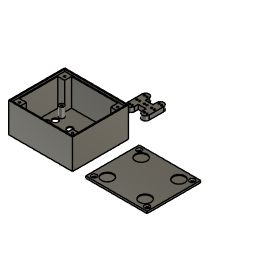
dice (Autodesk Fusion 360 design; units mm, degrees)
Autodesk Fusion 360 part; units mm, degrees
note: some values were not read from the file. Set by a fixed rule: which face or edge a step refers to.
sketch "Sketch1" plane through (0, 0, 0) normal (0, 0, 1) x (1, 0, 0)
  line L0 (0, 0) -> (61, 0)
  line L1 (61, 0) -> (61, -53)
  line L2 (61, -53) -> (0, -53)
  line L3 (0, -53) -> (0, 0)
  line L4 (-1, 1) -> (62, 1)
  line L5 (62, 1) -> (62, -54)
  line L6 (62, -54) -> (-1, -54)
  line L7 (-1, -54) -> (-1, 1)
  line L8 (-2, 2) -> (63, 2)
  line L9 (63, 2) -> (63, -55)
  line L10 (63, -55) -> (-2, -55)
  line L11 (-2, -55) -> (-2, 2)
  line L12 (0, -53) -> (7, -53)
  line L13 (7, -53) -> (7, -46)
  line L14 (7, -46) -> (0, -46)
  line L15 (0, -46) -> (0, -53)
  line L16 (61, -53) -> (54, -53)
  line L17 (54, -53) -> (54, -46)
  line L18 (54, -46) -> (61, -46)
  line L19 (61, -46) -> (61, -53)
  line L20 (61, 0) -> (54, 0)
  line L21 (54, 0) -> (54, -7)
  line L22 (54, -7) -> (61, -7)
  line L23 (61, -7) -> (61, 0)
  line L24 (0, 0) -> (7, 0)
  line L25 (7, 0) -> (7, -7)
  line L26 (7, -7) -> (0, -7)
  line L27 (0, -7) -> (0, 0)
  line L28 (61, 0) -> (53.5, 0)
  line L29 (61, -26.5) -> (61, 0)
  line L30 (61, 0) -> (43.5, 0)
  line L31 (61, -26.5) -> (61, 0)
  circle A0 centre (43.5, -26.5) radius 4
  circle A1 centre (53.5, -26.5) radius 3.5
  line L32 (61, -53) -> (42.5, -53)
  line L33 (61, -34.5) -> (61, -53)
  circle A2 centre (42.5, -34.5) radius 2.5
  line L34 (0, -53) -> (16.5, -53)
  line L35 (0, -34.5) -> (0, -53)
  circle A3 centre (16.5, -34.5) radius 2.5
  line L36 (0, 0) -> (9.5, 0)
  line L37 (0, -12.5) -> (0, 0)
  circle A4 centre (9.5, -12.5) radius 2.5
  line L38 (61, 0) -> (55.5, 0)
  line L39 (61, -19.5) -> (61, 0)
  circle A5 centre (55.5, -19.5) radius 2.5
  line L40 (0, 0) -> (9.5, 0)
  line L41 (0, -26.5) -> (0, 0)
  circle A6 centre (9.5, -19) radius 3
  circle A7 centre (9.5, -26.5) radius 3
  circle A8 centre (9.5, -34) radius 3
  circle A9 centre (17, -26.5) radius 3
  circle A10 centre (24.5, -19) radius 3
  circle A11 centre (24.5, -26.5) radius 3
  circle A12 centre (24.5, -34) radius 3
  dimension "d1" = 61
  dimension "d2" = 53
  dimension "d3" = 63
  dimension "d4" = 55
  dimension "d5" = 65
  dimension "d6" = 57
  dimension "d7" = 7
  dimension "d8" = 7
  dimension "d9" = 7
  dimension "d10" = 7
  dimension "d11" = 7
  dimension "d12" = 7
  dimension "d13" = 7
  dimension "d14" = 7
  dimension "d15" = 7.5
  dimension "d16" = 26.5
  dimension "d17" = 17.5
  dimension "d18" = 8
  dimension "d19" = 7
  dimension "d20" = 18.5
  dimension "d21" = 18.5
  dimension "d22" = 5
  dimension "d23" = 16.5
  dimension "d24" = 18.5
  dimension "d25" = 5
  dimension "d26" = 9.5
  dimension "d27" = 12.5
  dimension "d28" = 5
  dimension "d29" = 5.5
  dimension "d30" = 19.5
  dimension "d31" = 5
  dimension "d32" = 9.5
  dimension "d33" = 26.5
  dimension "d34" = 7.5
  dimension "d35" = 7.5
  dimension "d39" = 7.5
  dimension "d42" = 6
  dimension "d43" = 6
  dimension "d44" = 6
  dimension "d45" = 6
  dimension "d46" = 6
  dimension "d47" = 6
  dimension "d48" = 6
  constraint horizontal L0
  constraint vertical L1
  constraint horizontal L2
  constraint vertical L3
  constraint coincident L0.start L3.end
  constraint horizontal L4
  constraint vertical L5
  constraint horizontal L6
  constraint vertical L7
  constraint horizontal L8
  constraint vertical L9
  constraint horizontal L10
  constraint vertical L11
  constraint horizontal L12
  constraint vertical L13
  constraint horizontal L14
  constraint vertical L15
  constraint horizontal L16
  constraint vertical L17
  constraint horizontal L18
  constraint vertical L19
  constraint horizontal L20
  constraint vertical L21
  constraint horizontal L22
  constraint vertical L23
  constraint horizontal L24
  constraint vertical L25
  constraint horizontal L26
  constraint vertical L27
  constraint horizontal L28
  constraint vertical L29
  constraint horizontal L30
  constraint vertical L31
  constraint horizontal L32
  constraint vertical L33
  constraint horizontal L34
  constraint vertical L35
  constraint horizontal L36
  constraint vertical L37
  constraint horizontal L38
  constraint vertical L39
  constraint horizontal L40
  constraint vertical L41
  measures "d1" distance of L0.start L0.end
  measures "d2" distance of L0.start L2.end
  measures "d3" distance of L4.start L4.end
  measures "d4" distance of L4.start L6.end
  measures "d5" distance of L8.start L8.end
  measures "d6" distance of L8.start L10.end
  measures "d7" distance of L2.end L12.end
  measures "d8" distance of L2.end L14.end
  measures "d9" distance of L1.end L16.end
  measures "d10" distance of L1.end L18.end
  measures "d11" distance of L0.end L20.end
  measures "d12" distance of L0.end L22.end
  measures "d13" distance of L0.start L24.end
  measures "d14" distance of L0.start L26.end
  measures "d15" distance of L0.end L28.end
  measures "d16" distance of L0.end L29.start
  measures "d17" distance of L0.end L30.end
  measures "d18" diameter of A0
  measures "d19" diameter of A1
  measures "d20" distance of L1.end L32.end
  measures "d21" distance of L1.end L33.start
  measures "d22" diameter of A2
  measures "d23" distance of L2.end L34.end
  measures "d24" distance of L2.end L35.start
  measures "d25" diameter of A3
  measures "d26" distance of L0.start L36.end
  measures "d27" distance of L0.start L37.start
  measures "d28" diameter of A4
  measures "d29" distance of L0.end L38.end
  measures "d30" distance of L0.end L39.start
  measures "d31" diameter of A5
  measures "d32" distance of L0.start L36.end
  measures "d33" distance of L0.start L41.start
  measures "d34" distance of A7.centre A9.centre
  measures "d35" distance of A6.centre A7.centre
  measures "d39" distance of A7.centre A8.centre
  measures "d42" diameter of A6
  measures "d43" diameter of A7
  measures "d44" diameter of A8
  measures "d45" diameter of A9
  measures "d46" diameter of A10
  measures "d47" diameter of A11
  measures "d48" diameter of A12
extrude "Extrude1" add sketch "Sketch1" along normal blind 1 contours L0 L1 L2 L3 L13 L14 L17 L18 L21 L22 L25 L26 L28 L29 L30 L31 L32 L33 L34 L35 L36 L37 L39 L40 L41 makes body 1
extrude "Extrude2" add sketch "Sketch1" along normal blind 11 contours A2 | A3 | A4 | A5 bodies 1
extrude "Extrude3" add sketch "Sketch1" along normal blind 30 contours L0 L3 L24 L25 L26 L27 L36 L37 L40 L41 | L0 L1 L20 L21 L22 L23 L28 L29 L30 L31 L38 L39 | L2 L3 L12 L13 L14 L15 L34 L35 | L1 L2 L16 L17 L18 L19 L32 L33 | L4 L5 L6 L7 bodies 1
extrude "Extrude4" add sketch "Sketch1" along normal blind 31 contours L8 L9 L10 L11 bodies 1
sketch "Sketch2" plane through (0, 0, 11) normal (0, 0, 1) x (-1, 0, 0)
  circle A0 centre (-9.5, 12.5) radius 2.5
  circle A1 centre (-9.5, 12.5) radius 0.9
  circle A2 centre (-16.5, 34.5) radius 0.9
  circle A3 centre (-42.5, 34.5) radius 0.9
  circle A4 centre (-55.5, 19.5) radius 0.9
  dimension "d57" = 1.8
  dimension "d58" = 1.8
  dimension "d59" = 1.8
  dimension "d60" = 1.8
  constraint concentric A0 A1
  measures "d57" diameter of A1
  measures "d58" diameter of A2
  measures "d59" diameter of A3
  measures "d60" diameter of A4
extrude "Extrude5" cut sketch "Sketch2" against normal blind 7 contours A1 | A2 | A3 | A4 bodies 1
sketch "Sketch3" plane through (0, 0, 30) normal (0, 0, 1) x (-1, 0, 0)
  line L0 (0, 46) -> (0, 7)
  line L1 (0, 7) -> (-7, 7)
  line L2 (-7, 7) -> (-7, 0)
  line L3 (-7, 0) -> (-54, 0)
  line L4 (-54, 0) -> (-54, 7)
  line L5 (-54, 7) -> (-61, 7)
  line L6 (-61, 7) -> (-61, 46)
  line L7 (-61, 46) -> (-54, 46)
  line L8 (-54, 46) -> (-54, 53)
  line L9 (-54, 53) -> (-7, 53)
  line L10 (-7, 53) -> (-7, 46)
  line L11 (-7, 46) -> (0, 46)
  line L12 (1, 54) -> (-62, 54)
  line L13 (-62, 54) -> (-62, -1)
  line L14 (-62, -1) -> (1, -1)
  line L15 (1, -1) -> (1, 54)
  line L16 (1, -1) -> (-3.5, -1)
  line L17 (1, 3.5) -> (1, -1)
  circle A0 centre (-3.5, 3.5) radius 1
  line L18 (1, 54) -> (-3.5, 54)
  line L19 (1, 49.5) -> (1, 54)
  circle A1 centre (-3.5, 49.5) radius 1
  line L20 (-62, 54) -> (-57.5, 54)
  line L21 (-62, 49.5) -> (-62, 54)
  circle A2 centre (-57.5, 49.5) radius 1
  line L22 (-62, -1) -> (-57.5, -1)
  line L23 (-62, 3.5) -> (-62, -1)
  circle A3 centre (-57.5, 3.5) radius 1
  dimension "d63" = 2
  dimension "d64" = 4.5
  dimension "d65" = 4.5
  dimension "d66" = 2
  dimension "d67" = 4.5
  dimension "d68" = 4.5
  dimension "d69" = 2
  dimension "d70" = 4.5
  dimension "d71" = 4.5
  dimension "d72" = 2
  constraint horizontal L16
  constraint vertical L17
  constraint coincident L14.end L15.start
  constraint horizontal L18
  constraint vertical L19
  constraint coincident L12.start L15.end
  constraint horizontal L20
  constraint vertical L21
  constraint coincident L12.end L13.start
  constraint horizontal L22
  constraint vertical L23
  constraint coincident L13.end L14.start
  measures "d63" diameter of A0
  measures "d64" distance of L12.start L18.end
  measures "d65" distance of L12.start L19.start
  measures "d66" diameter of A1
  measures "d67" distance of L12.end L20.end
  measures "d68" distance of L12.end L21.start
  measures "d69" diameter of A2
  measures "d70" distance of L13.end L22.end
  measures "d71" distance of L13.end L23.start
  measures "d72" diameter of A3
extrude "Extrude6" cut sketch "Sketch3" against normal blind 12 contours A0 | A1 | A2 | A3 bodies 1
sketch "Sketch4" plane through (0, 0, 0) normal (0, 0, 1) x (1, 0, 0)
  line L0 (75, 1) -> (137.5, 1)
  line L1 (137.5, 1) -> (137.5, -53.5)
  line L2 (137.5, -53.5) -> (75, -53.5)
  line L3 (75, -53.5) -> (75, 1)
  line L4 (75, 1) -> (79.25, 1)
  line L5 (75, -3.25) -> (75, 1)
  circle A0 centre (79.25, -3.25) radius 1.4
  line L6 (75, -53.5) -> (79.25, -53.5)
  line L7 (75, -49.25) -> (75, -53.5)
  circle A1 centre (79.25, -49.25) radius 1.4
  line L8 (137.5, -53.5) -> (133.25, -53.5)
  line L9 (137.5, -49.25) -> (137.5, -53.5)
  circle A2 centre (133.25, -49.25) radius 1.4
  line L10 (137.5, 1) -> (133.25, 1)
  line L11 (137.5, -3.25) -> (137.5, 1)
  circle A3 centre (133.25, -3.25) radius 1.4
  line L12 (75, 1) -> (87, 1)
  line L13 (75, -9) -> (75, 1)
  line L14 (137.5, 1) -> (125.5, 1)
  line L15 (137.5, -9) -> (137.5, 1)
  line L16 (137.5, -53.5) -> (125.5, -53.5)
  line L17 (137.5, -43.5) -> (137.5, -53.5)
  line L18 (75, -53.5) -> (87, -53.5)
  line L19 (75, -43.5) -> (75, -53.5)
  dimension "d75" = 62.5
  dimension "d76" = 54.5
  dimension "d83" = 4.25
  dimension "d84" = 4.25
  dimension "d85" = 2.8
  dimension "d86" = 4.25
  dimension "d87" = 4.25
  dimension "d88" = 2.8
  dimension "d89" = 4.25
  dimension "d90" = 4.25
  dimension "d91" = 2.8
  dimension "d92" = 4.25
  dimension "d93" = 4.25
  dimension "d94" = 2.8
  constraint horizontal L0
  constraint vertical L1
  constraint horizontal L2
  constraint vertical L3
  constraint horizontal L4
  constraint vertical L5
  constraint horizontal L6
  constraint vertical L7
  constraint horizontal L8
  constraint vertical L9
  constraint horizontal L10
  constraint vertical L11
  constraint horizontal L12
  constraint vertical L13
  constraint horizontal L14
  constraint vertical L15
  constraint horizontal L16
  constraint vertical L17
  constraint horizontal L18
  constraint vertical L19
  measures "d75" distance of L0.start L0.end
  measures "d76" distance of L0.start L2.end
  measures "d83" distance of L0.start L4.end
  measures "d84" distance of L0.start L5.start
  measures "d85" diameter of A0
  measures "d86" distance of L2.end L6.end
  measures "d87" distance of L2.end L7.start
  measures "d88" diameter of A1
  measures "d89" distance of L1.end L8.end
  measures "d90" distance of L1.end L9.start
  measures "d91" diameter of A2
  measures "d92" distance of L0.end L10.end
  measures "d93" distance of L0.end L11.start
  measures "d94" diameter of A3
extrude "Extrude7" cut 1 faces at (3.1391, -0.5011, 30) along direction (0, 0, -1) blind 1 on bodies 1 bodies 1
extrude "Extrude8" add sketch "Sketch1" along normal blind 30 contours L4 L5 L6 L7 bodies 1
extrude "Extrude9" add 4 faces at (3.4751, -0.8343, 29) (57.5249, -6.1657, 29) (57.5249, -52.1657, 29) (3.5249, -52.1657, 29) along direction (0, 0, 1) blind 1 on bodies 1 bodies 1
extrude "Extrude10" cut 1 faces at (3.1391, -0.5011, 30) along direction (0, 0, -1) blind 1 on bodies 1 bodies 1
extrude "Extrude11" add sketch "Sketch4" along normal blind 2 separate body makes body 2
chamfer "Chamfer1" distance 1.2 angle 45 4 edges at (77.9447, -2.7437, 2) (77.9447, -48.7437, 2) (131.9447, -48.7437, 2) (131.9447, -2.7437, 2) on bodies 2
sketch "Sketch5" plane through (0, 0, 2) normal (0, 0, 1) x (-1, 0, 0)
  circle A0 centre (-133.25, 49.25) radius 2.6
  circle A1 centre (-79.25, 3.25) radius 2.6
  line L0 (-75, -1) -> (-75, 53.5)
  line L1 (-75, 53.5) -> (-137.5, 53.5)
  line L2 (-137.5, 53.5) -> (-137.5, -1)
  line L3 (-137.5, -1) -> (-75, -1)
  circle A2 centre (-79.25, 49.25) radius 2.6
  circle A3 centre (-133.25, 3.25) radius 2.6
  line L4 (-75, -1) -> (-87, -1)
  line L5 (-75, 9) -> (-75, -1)
  circle A4 centre (-87, 9) radius 6
  line L6 (-137.5, -1) -> (-125.5, -1)
  line L7 (-137.5, 9) -> (-137.5, -1)
  circle A5 centre (-125.5, 9) radius 6
  line L8 (-137.5, 53.5) -> (-125.5, 53.5)
  line L9 (-137.5, 43.5) -> (-137.5, 53.5)
  circle A6 centre (-125.5, 43.5) radius 6
  line L10 (-75, 53.5) -> (-87, 53.5)
  line L11 (-75, 43.5) -> (-75, 53.5)
  circle A7 centre (-87, 43.5) radius 6
  dimension "d114" = 12
  dimension "d115" = 10
  dimension "d116" = 12
  dimension "d117" = 12
  dimension "d118" = 10
  dimension "d119" = 12
  dimension "d120" = 12
  dimension "d121" = 10
  dimension "d122" = 12
  dimension "d123" = 12
  dimension "d124" = 10
  dimension "d125" = 12
  constraint horizontal L4
  constraint vertical L5
  constraint coincident L0.start L3.end
  constraint horizontal L6
  constraint vertical L7
  constraint coincident L2.end L3.start
  constraint horizontal L8
  constraint vertical L9
  constraint coincident L1.end L2.start
  constraint horizontal L10
  constraint vertical L11
  constraint coincident L0.end L1.start
  measures "d114" distance of L0.start L4.end
  measures "d115" distance of L0.start L5.start
  measures "d116" diameter of A4
  measures "d117" distance of L2.end L6.end
  measures "d118" distance of L2.end L7.start
  measures "d119" diameter of A5
  measures "d120" distance of L1.end L8.end
  measures "d121" distance of L1.end L9.start
  measures "d122" diameter of A6
  measures "d123" distance of L0.end L10.end
  measures "d124" distance of L0.end L11.start
  measures "d125" diameter of A7
extrude "Extrude12" cut sketch "Sketch5" against normal blind 0.8 contours A4 | A5 | A6 | A7 bodies 2
sketch "Sketch6" plane through (0, 0, 0) normal (0, 0, 1) x (1, 0, 0)
  circle A0 centre (5, 10) radius 3.5
  circle A1 centre (15, 10) radius 3
  dimension "d128" = 7
  dimension "d135" = 6
  measures "d128" diameter of A0
  measures "d135" diameter of A1
extrude "Extrude13" add sketch "Sketch6" along normal blind 8 separate body contours A0 makes body 3
sketch "Sketch7" plane through (0, 0, 8) normal (0, 0, 1) x (-1, 0, 0)
  circle A0 centre (-5, -10) radius 3.5
  circle A1 centre (-5, -10) radius 1.75
  dimension "d131" = 3.5
  constraint concentric A0 A1
  measures "d131" diameter of A1
extrude "Extrude15" add sketch "Sketch6" along normal blind 3.5 separate body contours A1 makes body 4
chamfer "Chamfer3" distance 0.6 angle 45 1 edges at (12.203, 8.9152, 0) on bodies 4
chamfer "Chamfer4" distance 0.6 angle 45 1 edges at (1.7369, 8.7343, 0) on bodies 3
sketch "Sketch8" plane through (0, 0, 3.5) normal (0, 0, 1) x (-1, 0, 0)
  circle A0 centre (-15, -10) radius 3
  line L0 (-13.3, -11.2) -> (-16.7, -11.2)
  line L1 (-16.7, -11.2) -> (-16.7, -8.8)
  line L2 (-16.7, -8.8) -> (-13.3, -8.8)
  line L3 (-13.3, -8.8) -> (-13.3, -11.2)
  dimension "d140" = 3.4
  dimension "d141" = 2.4
  constraint horizontal L0
  constraint vertical L1
  constraint horizontal L2
  constraint vertical L3
  measures "d140" distance of L0.start L0.end
  measures "d141" distance of L0.start L2.end
extrude "Extrude16" cut sketch "Sketch8" against normal blind 2.5 contours L0 L1 L2 L3 bodies 4
extrude "Extrude17" cut sketch "Sketch7" against normal blind 3.5 contours A1 bodies 3
chamfer "Chamfer5" distance 0.6 angle 45 4 edges at (30.5, 2, 0) (-2, -26.5, 0) (30.5, -55, 0) (63, -26.5, 0) on bodies 1
sketch "Sketch9" plane through (0, 0, 0) normal (0, 0, 1) x (1, 0, 0)
  circle A0 centre (37.5129, 45) radius 3
  circle A1 centre (37.5129, 37.5) radius 3
  circle A2 centre (37.5129, 30) radius 3
  circle A3 centre (45.0129, 37.5) radius 3
  circle A4 centre (52.5129, 37.5) radius 3
  circle A5 centre (52.5, 45) radius 3
  circle A6 centre (52.5, 30) radius 3
  circle A7 centre (37.5129, 45) radius 3.6
  circle A8 centre (37.5129, 37.5) radius 3.6
  circle A9 centre (37.5129, 30) radius 3.6
  circle A10 centre (45.0129, 37.5) radius 3.6
  circle A11 centre (52.5, 45) radius 3.6
  circle A12 centre (52.5129, 37.5) radius 3.6
  circle A13 centre (52.5, 30) radius 3.6
  line L0 (33.9129, 44.9997) -> (33.9129, 30)
  line L1 (48.9, 30.0018) -> (48.9, 33.9)
  line L2 (48.9, 33.9) -> (41.1129, 33.9)
  line L3 (41.1129, 33.9) -> (41.1129, 30.0018)
  line L4 (48.9, 45.0043) -> (48.9, 41.1)
  line L5 (48.9, 41.1) -> (41.1129, 41.1)
  line L6 (41.1129, 41.1) -> (41.1129, 45.0043)
  line L7 (56.1, 45) -> (56.1, 30)
  circle A14 centre (38.8, 45) radius 0.9
  circle A15 centre (36.2, 45) radius 0.9
  circle A16 centre (38.8, 37.5) radius 0.9
  circle A17 centre (36.2, 37.5) radius 0.9
  circle A18 centre (38.8, 30) radius 0.9
  circle A19 centre (36.2, 30) radius 0.9
  circle A20 centre (46.3, 37.5) radius 0.9
  circle A21 centre (43.7, 37.5) radius 0.9
  circle A22 centre (53.8, 45) radius 0.9
  circle A23 centre (51.2, 45) radius 0.9
  circle A24 centre (53.8, 37.5) radius 0.9
  circle A25 centre (51.2, 37.5) radius 0.9
  circle A26 centre (53.8, 30) radius 0.9
  circle A27 centre (51.2, 30) radius 0.9
  line L8 (34.6629, 49.5) -> (34.6629, 25)
  line L9 (42.1629, 42) -> (42.1629, 33)
  line L10 (49.65, 50) -> (49.65, 25)
  dimension "d147" = 6
  dimension "d148" = 6
  dimension "d149" = 7.5
  dimension "d150" = 6
  dimension "d151" = 7.5
  dimension "d152" = 6
  dimension "d153" = 7.5
  dimension "d154" = 7.5
  dimension "d155" = 6
  dimension "d156" = 7.5
  dimension "d157" = 7.5
  dimension "d158" = 6
  dimension "d159" = 6
  dimension "d160" = 7.2
  dimension "d161" = 7.2
  dimension "d162" = 7.2
  dimension "d163" = 7.2
  dimension "d164" = 7.2
  dimension "d165" = 7.2
  dimension "d166" = 7.2
  dimension "d167" = 1.8
  dimension "d168" = 1.8
  dimension "d169" = 2.6
  dimension "d170" = 1.8
  dimension "d171" = 1.8
  dimension "d172" = 1.8
  dimension "d173" = 1.8
  dimension "d174" = 1.8
  dimension "d175" = 1.8
  dimension "d176" = 1.8
  dimension "d177" = 1.8
  dimension "d178" = 1.8
  dimension "d179" = 1.8
  dimension "d180" = 1.8
  dimension "d181" = 1.8
  dimension "d182" = 2.85
  dimension "d183" = 2.85
  dimension "d184" = 14.9871
  dimension "d185" = 2.85
  constraint concentric A0 A7
  constraint concentric A1 A8
  constraint concentric A2 A9
  constraint concentric A3 A10
  constraint concentric A5 A11
  constraint concentric A4 A12
  constraint concentric A6 A13
  constraint coincident A7 L0.start
  constraint coincident A9 L0.end
  constraint tangent A9 L0
  constraint vertical L1
  constraint horizontal L2
  constraint vertical L3
  constraint coincident A9 L3.end
  constraint vertical L4
  constraint horizontal L5
  constraint vertical L6
  constraint coincident A7 L6.end
  constraint coincident A11 L7.start
  constraint coincident A13 L7.end
  constraint tangent A13 L7
  constraint parallel L0 L8
  constraint perpendicular L5 L9
  constraint vertical L10
  measures "d147" diameter of A0
  measures "d148" diameter of A1
  measures "d149" distance of A0.centre A1.centre
  measures "d150" diameter of A2
  measures "d151" distance of A1.centre A2.centre
  measures "d152" diameter of A3
  measures "d153" horizontal distance of A1.centre A3.centre
  measures "d154" vertical distance of A0.centre A3.centre
  measures "d155" diameter of A4
  measures "d156" horizontal distance of A3.centre A4.centre
  measures "d157" vertical distance of A0.centre A4.centre
  measures "d158" diameter of A5
  measures "d159" diameter of A6
  measures "d160" diameter of A7
  measures "d161" diameter of A8
  measures "d162" diameter of A9
  measures "d163" diameter of A10
  measures "d164" diameter of A11
  measures "d165" diameter of A12
  measures "d166" diameter of A13
  measures "d167" diameter of A14
  measures "d168" diameter of A15
  measures "d169" distance of A14.centre A15.centre
  measures "d170" diameter of A16
  measures "d171" diameter of A17
  measures "d172" diameter of A18
  measures "d173" diameter of A19
  measures "d174" diameter of A20
  measures "d175" diameter of A21
  measures "d176" diameter of A22
  measures "d177" diameter of A23
  measures "d178" diameter of A24
  measures "d179" diameter of A25
  measures "d180" diameter of A26
  measures "d181" diameter of A27
  measures "d182" distance of A0.centre L8
  measures "d183" distance of A3.centre L9
  measures "d184" distance of A5.centre A0.centre
  measures "d185" distance of A5.centre L10
extrude "Extrude18" add sketch "Sketch9" along normal blind 5.5 separate body contours A0 A7 L6 L8 | A0 L8 | A0 A7 L8 | A5 A11 L10 | A7 A8 L0 L8 | A7 A8 A9 A10 L2 L3 L5 L6 L8 L9 | A1 A8 L8 | A1 A8 L8 | A8 A9 L0 L8 | A1 L8 | A2 A9 L8 | A10 L5 L9 | A2 A9 L8 | A10 A11 A12 A13 L1 L2 L4 L5 L10 | A3 A10 L9 | A3 A10 L9 | A2 L8 | A10 L2 L9 | A3 L9 | A5 A11 L10 | A11 A12 L7 L10 | A6 A13 L10 | A5 L10 | A4 A12 L10 | A4 A12 L7 L10 | A12 A13 L7 L10 | A6 A13 L10 | A4 L10 | A6 L10 picked at (34.631, 45.1894) picked at (34.631, 37.6894) picked at (34.631, 30.1894) picked at (42.131, 37.6894) picked at (49.6181, 45.1894) picked at (49.6208, 37.6811) picked at (49.6181, 30.1894) makes body 5
extrude "Extrude19" add sketch "Sketch9" along normal blind 4.5 contours A0 L8 | A1 L8 | A2 L8 | A3 L9 | A5 L10 | A4 L10 | A6 L10 picked at (37.4402, 46.467) picked at (37.4402, 38.967) picked at (37.4402, 31.467) picked at (44.9402, 38.967) picked at (52.4359, 46.467) picked at (52.4321, 38.9665) picked at (52.4359, 31.467) bodies 5
extrude "Extrude20" cut 29 faces at (35.0073, 42.7118, 5.5) (34.631, 45.1894, 5.5) (34.1252, 45.2206, 5.5) (41.2636, 34.9047, 5.5) (34.4871, 40.7331, 5.5) (42.4877, 40.504, 5.5) (41.7707, 38.5016, 5.5) (42.4877, 34.496, 5.5) (35.0073, 32.2882, 5.5) (34.4871, 34.2669, 5.5) (35.0073, 39.7882, 5.5) (34.1252, 37.2792, 5.5) (45.268, 34.1158, 5.5) (42.131, 37.6894, 5.5) (34.1252, 29.7792, 5.5) (34.631, 37.6894, 5.5) (48.8638, 34.9237, 5.5) (34.631, 30.1894, 5.5) (49.1122, 44.7818, 5.5) (50.527, 41.0453, 5.5) (49.2645, 36.5178, 5.5) (50.527, 33.9547, 5.5) (49.1123, 29.7803, 5.5) (49.9944, 42.7118, 5.5) (49.6181, 45.1894, 5.5) (55.9043, 37.5, 5.5) (49.6208, 37.6811, 5.5) (49.9944, 32.2882, 5.5) (49.6181, 30.1894, 5.5) along direction (0, 0, -1) blind 1 on bodies 5 bodies 5
extrude "Extrude14" [suppressed]
chamfer "Chamfer2" [suppressed]
